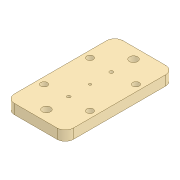
# Autodesk Inventor part: Inferior_base
Saved by Autodesk Inventor 2020 (Build 240168000, 168)
## iProperties
Created: 2022-07-20
Part Number: Inferior_base
Material: Genérico
Document SubType Name: Modeling
Designer: gabri
Density: 1 g/cm^3
Appearance: Bege
Author: gabri
Autodesk Inventor part; units mm, degrees
ref_plane "YZ Plane" through (0, 0, 0) normal (1, 0, 0) x (0, 1, 0)
ref_plane "XZ Plane" through (0, 0, 0) normal (0, 1, 0) x (-1, 0, 0)
ref_plane "XY Plane" through (0, 0, 0) normal (0, 0, 1) x (1, 0, 0)
sketch "Esboço1" plane through (0, 0, 0) normal (0, 1, 0) x (-1, 0, 0)
  circle A0 centre (0, 0) radius 34.95
  circle A1 centre (0, 0) radius 1.5
  line L0 (36, 66.1815) -> (-36, 66.1815)
  line L1 (-36, 66.1815) -> (-36, -66.1815)
  line L2 (-36, -66.1815) -> (36, -66.1815)
  line L3 (36, -66.1815) -> (36, 66.1815)
  line L4 (36, 66.1815) -> (-36, -66.1815) construction
  line L5 (-36, 66.1815) -> (36, -66.1815) construction
  dimension "d0" = 69.9
  dimension "d3" = 3
  dimension "d11" = 132.363
  dimension "d12" = 72
  constraints: 12 end point, 2 centre point, 2 coincident, 2 midpoint, 2 parallel, 1 horizontal, 1 perpendicular
  measures "d0" diameter of A0
  measures "d3" diameter of A1
  measures "d11" distance of L0.end L1.end
  measures "d12" distance of L1.end L2.end
extrude "Extrusão1" add sketch "Esboço1" along normal blind 12 contours A0 | L3 L2 L1 L0
sketch "Esboço2" plane through (0, 0, 0) normal (0, -1, 0) x (1, 0, 0)
  circle A0 centre (0, 0) radius 1.5 projected
  circle A1 centre (0, 0) radius 26
  circle A2 centre (0, -26) radius 2.1
  circle A3 centre (0, 26) radius 2.1
  circle A4 centre (0, 53.1) radius 5
  circle A5 centre (0, -53.1) radius 5
  dimension "d4" = 4.2
  dimension "d5" = 4.2
  dimension "d13" = 10
  dimension "d14" = 53.1
  dimension "d15" = 10
  dimension "d16" = 53.1
  dimension "d20" = 52
  constraints: 5 centre point, 2 point on circle, 1 coincident
  measures "d4" diameter of A2
  measures "d5" diameter of A3
  measures "d13" diameter of A4
  measures "d14" distance of point (0, 0) A4.centre
  measures "d15" diameter of A5
  measures "d16" distance of point (0, 0) A5.centre
  measures "d20" diameter of A1
extrude "Extrusão2" cut sketch "Esboço2" against normal blind 12 contours A3 A1 | A1 A3 | A2 A1 | A1 A2 | A4 | A5
chamfer "Chanfro1" distance 2.5 angle 45 2 edges at (-2.1, 0, 26) (-2.1, 0, -26)
fillet "Arredondamento1" radius 10 4 edges at (-36, 6, -66.1815) (36, 6, -66.1815) (36, 6, 66.1815) (-36, 6, 66.1815)
sketch "Esboço3" plane through (0, 0, 0) normal (0, -1, 0) x (1, 0, 0)
  circle A0 centre (28, -28) radius 4
  circle A1 centre (0, 0) radius 1.5 projected
  line L0 (0, 0) -> (13.6078, 0)
  line L1 (13.6078, 0) -> (13.6078, -9.8158)
  line L2 (13.6078, -9.8158) -> (0, -9.8158)
  line L3 (0, -9.8158) -> (0, 0)
  circle A2 centre (28, 28) radius 4
  circle A3 centre (-28, -28) radius 4
  circle A4 centre (-28, 28) radius 4
  dimension "d22" = 8
  dimension "d23" = 28
  dimension "d24" = 28
  dimension "d27" = 56
  dimension "d30" = 56
  constraints: 8 end point, 4 centre point, 2 horizontal, 2 parallel, 1 perpendicular, 1 vertical, 6 other
  measures "d22" diameter of A0
  measures "d23" horizontal distance of point (0, 0) A0.centre
  measures "d24" horizontal distance of point (0, 0) A0.centre
  measures "d27" distance of A0.centre A2.centre
  measures "d30" distance of A0.centre A3.centre
extrude "Extrusão3" cut sketch "Esboço3" against normal blind 12 contours A0 | A2 | A3 | A4
equation "\"d16\" = d14"
